Autodesk Fusion 360 part; units mm, degrees
(part 2 of 4)
  spline S9 degree 5 poles (-4.69563, -13.417878) (-4.69084, -13.420961) (-4.681355, -13.42726) (-4.667416, -13.437105) (-4.649379, -13.450989) (-4.627583, -13.469387) (-4.606332, -13.48855) (-4.58542, -13.508202) (-4.564695, -13.528137) (-4.544101, -13.548273) (-4.523643, -13.568609) (-4.503366, -13.589197) (-4.483326, -13.610104) (-4.463562, -13.631378) (-4.444078, -13.65302) (-4.424855, -13.675002) (-4.405861, -13.697281) (-4.387063, -13.71981) (-4.368435, -13.742557) (-4.349971, -13.765508) (-4.331672, -13.788665) (-4.313547, -13.812036) (-4.295604, -13.835631) (-4.27785, -13.859454) (-4.260283, -13.883502) (-4.242898, -13.907768) (-4.225689, -13.93224) (-4.208647, -13.956907) (-4.191769, -13.981763) (-4.175051, -14.006801) (-4.158495, -14.032021) (-4.1421, -14.057422) (-4.125867, -14.083003) (-4.109797, -14.108764) (-4.093889, -14.134702) (-4.078141, -14.160813) (-4.062552, -14.187093) (-4.047119, -14.213539) (-4.031842, -14.240149) (-4.016718, -14.266918) (-4.001749, -14.293845) (-3.986933, -14.32093) (-3.972271, -14.348169) (-3.957762, -14.375562) (-3.943405, -14.403106) (-3.9292, -14.4308) (-3.915146, -14.458641) (-3.901243, -14.486627) (-3.887491, -14.514757) (-3.873888, -14.543029) (-3.860434, -14.57144) (-3.84713, -14.599991) (-3.833974, -14.628678) (-3.820967, -14.657502) (-3.808109, -14.686459) (-3.795398, -14.715549) (-3.782836, -14.74477) (-3.770421, -14.774121) (-3.758153, -14.8036) (-3.746033, -14.833206) (-3.73406, -14.862938) (-3.722233, -14.892795) (-3.710553, -14.922775) (-3.69902, -14.952876) (-3.687633, -14.983098) (-3.676392, -15.01344) (-3.665298, -15.043899) (-3.65435, -15.074474) (-3.643548, -15.105165) (-3.632893, -15.135971) (-3.622383, -15.16689) (-3.614091, -15.191717) (-3.607937, -15.210388) (-3.603864, -15.222858) (-3.601835, -15.229098) knots 0 0 0 0 0 0 0.01428571 0.02857143 0.04285714 0.05714286 0.07142857 0.08571429 0.1 0.11428571 0.12857143 0.14285714 0.15714286 0.17142857 0.18571429 0.2 0.21428571 0.22857143 0.24285714 0.25714286 0.27142857 0.28571429 0.3 0.31428571 0.32857143 0.34285714 0.35714286 0.37142857 0.38571429 0.4 0.41428571 0.42857143 0.44285714 0.45714286 0.47142857 0.48571429 0.5 0.51428571 0.52857143 0.54285714 0.55714286 0.57142857 0.58571429 0.6 0.61428571 0.62857143 0.64285714 0.65714286 0.67142857 0.68571429 0.7 0.71428571 0.72857143 0.74285714 0.75714286 0.77142857 0.78571429 0.8 0.81428571 0.82857143 0.84285714 0.85714286 0.87142857 0.88571429 0.9 0.91428571 0.92857143 0.94285714 0.95714286 0.97142857 0.98571429 1 1 1 1 1 1
  line L9 (-4.69563, -13.417878) -> (-4.967876, -13.242652)
  line L10 (-4.547342, -12.508165) -> (-4.258409, -12.654246)
  spline S10 degree 5 poles (-4.258409, -12.654246) (-4.253325, -12.656816) (-4.243091, -12.661807) (-4.227544, -12.668844) (-4.20644, -12.677371) (-4.17954, -12.686854) (-4.152256, -12.69548) (-4.124722, -12.703566) (-4.097038, -12.711347) (-4.069248, -12.718915) (-4.041354, -12.726263) (-4.013334, -12.733327) (-3.985159, -12.740026) (-3.956807, -12.746301) (-3.92828, -12.752148) (-3.899591, -12.757598) (-3.870763, -12.7627) (-3.841817, -12.767507) (-3.81277, -12.772056) (-3.78363, -12.776361) (-3.754396, -12.780419) (-3.725065, -12.784219) (-3.695634, -12.787748) (-3.666102, -12.791) (-3.636469, -12.793975) (-3.606742, -12.796684) (-3.576926, -12.799137) (-3.547025, -12.801346) (-3.517046, -12.80332) (-3.48699, -12.805062) (-3.456859, -12.806573) (-3.426653, -12.807854) (-3.396374, -12.808902) (-3.366023, -12.80972) (-3.335602, -12.810309) (-3.305112, -12.810672) (-3.274556, -12.810812) (-3.243936, -12.810733) (-3.213254, -12.810438) (-3.182513, -12.809929) (-3.151712, -12.809207) (-3.120855, -12.808273) (-3.089941, -12.807129) (-3.058973, -12.805775) (-3.027951, -12.804212) (-2.996877, -12.802443) (-2.965752, -12.800469) (-2.934579, -12.798291) (-2.903358, -12.795912) (-2.87209, -12.793331) (-2.840777, -12.79055) (-2.80942, -12.787571) (-2.77802, -12.784394) (-2.746578, -12.78102) (-2.715096, -12.77745) (-2.683575, -12.773685) (-2.652015, -12.769726) (-2.620418, -12.765575) (-2.588785, -12.761231) (-2.557117, -12.756696) (-2.525415, -12.751971) (-2.49368, -12.747056) (-2.461913, -12.741952) (-2.430114, -12.73666) (-2.398286, -12.731181) (-2.36643, -12.725515) (-2.334546, -12.719663) (-2.302635, -12.713626) (-2.270699, -12.707405) (-2.238738, -12.701) (-2.206753, -12.694411) (-2.181145, -12.688994) (-2.161928, -12.684849) (-2.149112, -12.682049) (-2.142703, -12.68064) knots 0 0 0 0 0 0 0.01428571 0.02857143 0.04285714 0.05714286 0.07142857 0.08571429 0.1 0.11428571 0.12857143 0.14285714 0.15714286 0.17142857 0.18571429 0.2 0.21428571 0.22857143 0.24285714 0.25714286 0.27142857 0.28571429 0.3 0.31428571 0.32857143 0.34285714 0.35714286 0.37142857 0.38571429 0.4 0.41428571 0.42857143 0.44285714 0.45714286 0.47142857 0.48571429 0.5 0.51428571 0.52857143 0.54285714 0.55714286 0.57142857 0.58571429 0.6 0.61428571 0.62857143 0.64285714 0.65714286 0.67142857 0.68571429 0.7 0.71428571 0.72857143 0.74285714 0.75714286 0.77142857 0.78571429 0.8 0.81428571 0.82857143 0.84285714 0.85714286 0.87142857 0.88571429 0.9 0.91428571 0.92857143 0.94285714 0.95714286 0.97142857 0.98571429 1 1 1 1 1 1
  arc A5 (-2.142703, -12.68064) -> (-1.961546, -12.203578) centre (-12.332883, -8.53815) ccw
  spline S11 degree 5 poles (-3.561505, -10.819006) (-3.555996, -10.820458) (-3.545029, -10.823518) (-3.52873, -10.828574) (-3.507285, -10.836204) (-3.480872, -10.846966) (-3.454739, -10.858624) (-3.428777, -10.870852) (-3.402906, -10.883408) (-3.377098, -10.896194) (-3.351357, -10.909213) (-3.32571, -10.922527) (-3.30019, -10.936218) (-3.27482, -10.950344) (-3.249602, -10.964906) (-3.224527, -10.979871) (-3.199578, -10.99519) (-3.174738, -11.010808) (-3.149993, -11.026685) (-3.12534, -11.042808) (-3.100781, -11.059177) (-3.07632, -11.075803) (-3.051965, -11.092698) (-3.027718, -11.109869) (-3.00358, -11.127312) (-2.979547, -11.145017) (-2.955618, -11.162973) (-2.931787, -11.181168) (-2.908054, -11.199591) (-2.884418, -11.218238) (-2.860878, -11.237107) (-2.837436, -11.256198) (-2.814093, -11.275512) (-2.790849, -11.295046) (-2.767704, -11.314798) (-2.744659, -11.334764) (-2.721711, -11.354941) (-2.698861, -11.375324) (-2.676109, -11.39591) (-2.653454, -11.416696) (-2.630896, -11.43768) (-2.608436, -11.45886) (-2.586074, -11.480235) (-2.56381, -11.501804) (-2.541644, -11.523563) (-2.519576, -11.545512) (-2.497607, -11.567648) (-2.475737, -11.589968) (-2.453964, -11.612471) (-2.432291, -11.635156) (-2.410716, -11.658019) (-2.38924, -11.681061) (-2.367863, -11.704279) (-2.346586, -11.727673) (-2.325409, -11.751239) (-2.304331, -11.774978) (-2.283354, -11.798887) (-2.262476, -11.822965) (-2.2417, -11.84721) (-2.221024, -11.871622) (-2.200449, -11.896199) (-2.179975, -11.920939) (-2.159602, -11.945842) (-2.139332, -11.970907) (-2.119163, -11.996131) (-2.099096, -12.021514) (-2.079133, -12.047054) (-2.059272, -12.07275) (-2.039515, -12.098601) (-2.019862, -12.124606) (-2.000311, -12.150764) (-1.984754, -12.171813) (-1.973132, -12.187669) (-1.965404, -12.19827) (-1.961546, -12.203578) knots 0 0 0 0 0 0 0.01428571 0.02857143 0.04285714 0.05714286 0.07142857 0.08571429 0.1 0.11428571 0.12857143 0.14285714 0.15714286 0.17142857 0.18571429 0.2 0.21428571 0.22857143 0.24285714 0.25714286 0.27142857 0.28571429 0.3 0.31428571 0.32857143 0.34285714 0.35714286 0.37142857 0.38571429 0.4 0.41428571 0.42857143 0.44285714 0.45714286 0.47142857 0.48571429 0.5 0.51428571 0.52857143 0.54285714 0.55714286 0.57142857 0.58571429 0.6 0.61428571 0.62857143 0.64285714 0.65714286 0.67142857 0.68571429 0.7 0.71428571 0.72857143 0.74285714 0.75714286 0.77142857 0.78571429 0.8 0.81428571 0.82857143 0.84285714 0.85714286 0.87142857 0.88571429 0.9 0.91428571 0.92857143 0.94285714 0.95714286 0.97142857 0.98571429 1 1 1 1 1 1
  line L11 (-3.561505, -10.819006) -> (-3.874574, -10.736485)
  line L12 (-3.701592, -9.907995) -> (-3.381658, -9.95764)
  spline S12 degree 5 poles (-3.381658, -9.95764) (-3.376029, -9.958513) (-3.364753, -9.960098) (-3.347793, -9.961986) (-3.325087, -9.963574) (-3.296573, -9.96428) (-3.267959, -9.964053) (-3.239273, -9.963235) (-3.21054, -9.96208) (-3.181772, -9.96069) (-3.152972, -9.959058) (-3.12414, -9.957119) (-3.095274, -9.954783) (-3.066371, -9.951989) (-3.037433, -9.948735) (-3.008465, -9.945053) (-2.979471, -9.940997) (-2.950456, -9.936624) (-2.921425, -9.931975) (-2.892381, -9.927064) (-2.863323, -9.921889) (-2.834254, -9.91644) (-2.805173, -9.910702) (-2.776081, -9.904668) (-2.74698, -9.898341) (-2.71787, -9.891731) (-2.688755, -9.88485) (-2.659636, -9.877711) (-2.630513, -9.870324) (-2.60139, -9.862693) (-2.572267, -9.854819) (-2.543144, -9.846703) (-2.514023, -9.838344) (-2.484905, -9.829743) (-2.45579, -9.820902) (-2.42668, -9.811825) (-2.397577, -9.802516) (-2.36848, -9.792979) (-2.339391, -9.783217) (-2.310311, -9.773233) (-2.281242, -9.763029) (-2.252183, -9.752605) (-2.223136, -9.741964) (-2.194101, -9.731106) (-2.165081, -9.720034) (-2.136074, -9.708749) (-2.107083, -9.697254) (-2.078108, -9.685549) (-2.049151, -9.673638) (-2.020211, -9.661522) (-1.99129, -9.649201) (-1.962388, -9.636678) (-1.933507, -9.623953) (-1.904647, -9.611028) (-1.875808, -9.597904) (-1.846993, -9.584583) (-1.818201, -9.571065) (-1.789434, -9.557353) (-1.760691, -9.543447) (-1.731975, -9.529348) (-1.703284, -9.515057) (-1.674621, -9.500576) (-1.645986, -9.485906) (-1.617379, -9.471046) (-1.588802, -9.456) (-1.560256, -9.440767) (-1.531741, -9.425349) (-1.503257, -9.409747) (-1.474807, -9.393961) (-1.44639, -9.377993) (-1.418006, -9.361843) (-1.395325, -9.348778) (-1.37833, -9.338897) (-1.367006, -9.332274) (-1.361346, -9.328954) knots 0 0 0 0 0 0 0.01428571 0.02857143 0.04285714 0.05714286 0.07142857 0.08571429 0.1 0.11428571 0.12857143 0.14285714 0.15714286 0.17142857 0.18571429 0.2 0.21428571 0.22857143 0.24285714 0.25714286 0.27142857 0.28571429 0.3 0.31428571 0.32857143 0.34285714 0.35714286 0.37142857 0.38571429 0.4 0.41428571 0.42857143 0.44285714 0.45714286 0.47142857 0.48571429 0.5 0.51428571 0.52857143 0.54285714 0.55714286 0.57142857 0.58571429 0.6 0.61428571 0.62857143 0.64285714 0.65714286 0.67142857 0.68571429 0.7 0.71428571 0.72857143 0.74285714 0.75714286 0.77142857 0.78571429 0.8 0.81428571 0.82857143 0.84285714 0.85714286 0.87142857 0.88571429 0.9 0.91428571 0.92857143 0.94285714 0.95714286 0.97142857 0.98571429 1 1 1 1 1 1
  arc A6 (-1.361346, -9.328954) -> (-1.336476, -8.819259) centre (-12.332883, -8.53815) ccw
  spline S13 degree 5 poles (-3.285983, -7.996868) (-3.280296, -7.996547) (-3.26892, -7.996068) (-3.251856, -7.995839) (-3.229103, -7.99647) (-3.200656, -7.998543) (-3.1722, -8.001555) (-3.14373, -8.005162) (-3.115246, -8.009108) (-3.086749, -8.013293) (-3.058246, -8.01772) (-3.02974, -8.022458) (-3.001238, -8.027593) (-2.972744, -8.033187) (-2.944261, -8.039244) (-2.915788, -8.045728) (-2.887327, -8.052588) (-2.858876, -8.059765) (-2.830436, -8.067218) (-2.802007, -8.074933) (-2.773592, -8.082912) (-2.745191, -8.091166) (-2.716807, -8.099708) (-2.688441, -8.108546) (-2.660093, -8.117676) (-2.631766, -8.127088) (-2.603458, -8.136771) (-2.575172, -8.146711) (-2.546908, -8.156898) (-2.518666, -8.167329) (-2.490447, -8.178) (-2.462253, -8.188913) (-2.434084, -8.200068) (-2.405942, -8.211463) (-2.377826, -8.223096) (-2.349738, -8.234964) (-2.321679, -8.247062) (-2.293649, -8.259387) (-2.265649, -8.271934) (-2.237679, -8.284702) (-2.209741, -8.297688) (-2.181835, -8.310891) (-2.153962, -8.32431) (-2.126123, -8.337942) (-2.098318, -8.351787) (-2.070548, -8.365843) (-2.042814, -8.380106) (-2.015116, -8.394576) (-1.987456, -8.409249) (-1.959833, -8.424126) (-1.932249, -8.439204) (-1.904704, -8.454481) (-1.877198, -8.469958) (-1.849734, -8.485631) (-1.82231, -8.5015) (-1.794928, -8.517563) (-1.767589, -8.53382) (-1.740294, -8.550268) (-1.713042, -8.566906) (-1.685834, -8.583734) (-1.658671, -8.60075) (-1.631554, -8.617952) (-1.604483, -8.635341) (-1.577459, -8.652915) (-1.550483, -8.670672) (-1.523555, -8.688612) (-1.496676, -8.706733) (-1.469847, -8.725034) (-1.443069, -8.743514) (-1.416341, -8.762173) (-1.389664, -8.78101) (-1.368363, -8.796221) (-1.352411, -8.807709) (-1.341786, -8.815403) (-1.336476, -8.819259) knots 0 0 0 0 0 0 0.01428571 0.02857143 0.04285714 0.05714286 0.07142857 0.08571429 0.1 0.11428571 0.12857143 0.14285714 0.15714286 0.17142857 0.18571429 0.2 0.21428571 0.22857143 0.24285714 0.25714286 0.27142857 0.28571429 0.3 0.31428571 0.32857143 0.34285714 0.35714286 0.37142857 0.38571429 0.4 0.41428571 0.42857143 0.44285714 0.45714286 0.47142857 0.48571429 0.5 0.51428571 0.52857143 0.54285714 0.55714286 0.57142857 0.58571429 0.6 0.61428571 0.62857143 0.64285714 0.65714286 0.67142857 0.68571429 0.7 0.71428571 0.72857143 0.74285714 0.75714286 0.77142857 0.78571429 0.8 0.81428571 0.82857143 0.84285714 0.85714286 0.87142857 0.88571429 0.9 0.91428571 0.92857143 0.94285714 0.95714286 0.97142857 0.98571429 1 1 1 1 1 1
  line L13 (-3.285983, -7.996868) -> (-3.60923, -8.015129)
  line L14 (-3.700732, -7.173734) -> (-3.381116, -7.122084)
  spline S14 degree 5 poles (-3.381116, -7.122084) (-3.375492, -7.121176) (-3.364279, -7.119198) (-3.347565, -7.115753) (-3.325479, -7.110246) (-3.298143, -7.102107) (-3.270999, -7.093049) (-3.243971, -7.083406) (-3.217, -7.073429) (-3.19007, -7.063217) (-3.163184, -7.052766) (-3.136363, -7.042011) (-3.109631, -7.03087) (-3.083006, -7.019281) (-3.05649, -7.007244) (-3.030077, -6.99479) (-3.003756, -6.981973) (-2.977513, -6.968848) (-2.951339, -6.955456) (-2.925234, -6.94181) (-2.899198, -6.927909) (-2.873235, -6.913744) (-2.847351, -6.8993) (-2.821547, -6.884571) (-2.795825, -6.869561) (-2.770183, -6.85428) (-2.744619, -6.838738) (-2.719131, -6.822951) (-2.693717, -6.806926) (-2.668377, -6.790668) (-2.643112, -6.77418) (-2.617923, -6.757462) (-2.59281, -6.740513) (-2.567775, -6.723335) (-2.542817, -6.70593) (-2.517937, -6.688302) (-2.493134, -6.670455) (-2.468409, -6.652393) (-2.44376, -6.634121) (-2.419189, -6.615639) (-2.394695, -6.596951) (-2.37028, -6.578058) (-2.345943, -6.558961) (-2.321685, -6.539663) (-2.297506, -6.520165) (-2.273406, -6.500469) (-2.249387, -6.480577) (-2.225447, -6.460492) (-2.201587, -6.440215) (-2.177808, -6.419749) (-2.15411, -6.399094) (-2.130492, -6.378253) (-2.106957, -6.357226) (-2.083503, -6.336015) (-2.060132, -6.314622) (-2.036843, -6.293049) (-2.013638, -6.271295) (-1.990516, -6.249365) (-1.967477, -6.227257) (-1.944523, -6.204974) (-1.921653, -6.182517) (-1.898868, -6.159888) (-1.876167, -6.137086) (-1.853553, -6.114114) (-1.831024, -6.090974) (-1.808582, -6.067665) (-1.786226, -6.04419) (-1.763959, -6.020549) (-1.741779, -5.996745) (-1.719687, -5.972777) (-1.697682, -5.948646) (-1.680149, -5.929212) (-1.667039, -5.914563) (-1.658316, -5.904765) (-1.653959, -5.899857) knots 0 0 0 0 0 0 0.01428571 0.02857143 0.04285714 0.05714286 0.07142857 0.08571429 0.1 0.11428571 0.12857143 0.14285714 0.15714286 0.17142857 0.18571429 0.2 0.21428571 0.22857143 0.24285714 0.25714286 0.27142857 0.28571429 0.3 0.31428571 0.32857143 0.34285714 0.35714286 0.37142857 0.38571429 0.4 0.41428571 0.42857143 0.44285714 0.45714286 0.47142857 0.48571429 0.5 0.51428571 0.52857143 0.54285714 0.55714286 0.57142857 0.58571429 0.6 0.61428571 0.62857143 0.64285714 0.65714286 0.67142857 0.68571429 0.7 0.71428571 0.72857143 0.74285714 0.75714286 0.77142857 0.78571429 0.8 0.81428571 0.82857143 0.84285714 0.85714286 0.87142857 0.88571429 0.9 0.91428571 0.92857143 0.94285714 0.95714286 0.97142857 0.98571429 1 1 1 1 1 1
  arc A7 (-1.653959, -5.899857) -> (-1.78781, -5.407424) centre (-12.332883, -8.53815) ccw
  spline S15 degree 5 poles (-3.896035, -5.227714) (-3.890725, -5.225651) (-3.880054, -5.22168) (-3.863896, -5.21619) (-3.842062, -5.209759) (-3.814367, -5.20294) (-3.786373, -5.197011) (-3.758182, -5.191644) (-3.729872, -5.186595) (-3.701477, -5.181769) (-3.673, -5.177171) (-3.644426, -5.172868) (-3.615732, -5.168944) (-3.586904, -5.16546) (-3.557943, -5.162418) (-3.52886, -5.159787) (-3.499672, -5.157515) (-3.470396, -5.155549) (-3.441044, -5.153849) (-3.411623, -5.152402) (-3.382133, -5.15121) (-3.352572, -5.150283) (-3.322937, -5.149636) (-3.293228, -5.149275) (-3.263447, -5.149199) (-3.233597, -5.149397) (-3.203683, -5.149858) (-3.17371, -5.150571) (-3.143681, -5.151525) (-3.113598, -5.152718) (-3.083463, -5.154147) (-3.053276, -5.155814) (-3.023039, -5.157717) (-2.992753, -5.159858) (-2.962418, -5.162234) (-2.932038, -5.164842) (-2.901613, -5.167677) (-2.871147, -5.170736) (-2.840639, -5.174017) (-2.810093, -5.177517) (-2.77951, -5.181234) (-2.74889, -5.185167) (-2.718234, -5.189316) (-2.687545, -5.193679) (-2.656822, -5.198254) (-2.626068, -5.20304) (-2.595284, -5.208035) (-2.56447, -5.213237) (-2.533629, -5.218645) (-2.502761, -5.224258) (-2.471868, -5.230074) (-2.44095, -5.236092) (-2.410008, -5.242311) (-2.379045, -5.24873) (-2.34806, -5.255348) (-2.317054, -5.262164) (-2.28603, -5.269176) (-2.254987, -5.276384) (-2.223927, -5.283787) (-2.192851, -5.291384) (-2.16176, -5.299173) (-2.130654, -5.307154) (-2.099535, -5.315326) (-2.068403, -5.323689) (-2.037259, -5.332241) (-2.006106, -5.340981) (-1.974943, -5.349909) (-1.943772, -5.359024) (-1.912593, -5.368325) (-1.881408, -5.377812) (-1.850216, -5.387483) (-1.825257, -5.395367) (-1.806535, -5.401363) (-1.794052, -5.405398) (-1.78781, -5.407424) knots 0 0 0 0 0 0 0.01428571 0.02857143 0.04285714 0.05714286 0.07142857 0.08571429 0.1 0.11428571 0.12857143 0.14285714 0.15714286 0.17142857 0.18571429 0.2 0.21428571 0.22857143 0.24285714 0.25714286 0.27142857 0.28571429 0.3 0.31428571 0.32857143 0.34285714 0.35714286 0.37142857 0.38571429 0.4 0.41428571 0.42857143 0.44285714 0.45714286 0.47142857 0.48571429 0.5 0.51428571 0.52857143 0.54285714 0.55714286 0.57142857 0.58571429 0.6 0.61428571 0.62857143 0.64285714 0.65714286 0.67142857 0.68571429 0.7 0.71428571 0.72857143 0.74285714 0.75714286 0.77142857 0.78571429 0.8 0.81428571 0.82857143 0.84285714 0.85714286 0.87142857 0.88571429 0.9 0.91428571 0.92857143 0.94285714 0.95714286 0.97142857 0.98571429 1 1 1 1 1 1
  line L15 (-3.896035, -5.227714) -> (-4.197818, -5.344971)
  line L16 (-4.544847, -4.573032) -> (-4.256835, -4.425143)
  spline S16 degree 5 poles (-4.256835, -4.425143) (-4.251767, -4.422541) (-4.241714, -4.417195) (-4.226882, -4.408754) (-4.207579, -4.396692) (-4.184097, -4.380504) (-4.16108, -4.363501) (-4.138354, -4.345978) (-4.115787, -4.328155) (-4.09333, -4.31012) (-4.07099, -4.291873) (-4.048805, -4.273357) (-4.026824, -4.2545) (-4.005083, -4.235251) (-3.983585, -4.215609) (-3.962313, -4.195603) (-3.941241, -4.175279) (-3.920338, -4.154687) (-3.899584, -4.133862) (-3.878973, -4.112817) (-3.858507, -4.091551) (-3.838192, -4.070056) (-3.818038, -4.04832) (-3.798049, -4.026339) (-3.778224, -4.004115) (-3.758559, -3.981657) (-3.739049, -3.958977) (-3.719687, -3.936086) (-3.700469, -3.912992) (-3.681393, -3.8897) (-3.66246, -3.866211) (-3.64367, -3.842527) (-3.625024, -3.818648) (-3.606522, -3.794574) (-3.588164, -3.770308) (-3.569949, -3.745855) (-3.551875, -3.721217) (-3.533941, -3.696399) (-3.516146, -3.671403) (-3.498488, -3.646234) (-3.480968, -3.620891) (-3.463586, -3.595378) (-3.446341, -3.569696) (-3.429234, -3.543845) (-3.412264, -3.51783) (-3.39543, -3.491651) (-3.378733, -3.46531) (-3.362171, -3.43881) (-3.345745, -3.412153) (-3.329455, -3.38534) (-3.313299, -3.358373) (-3.297278, -3.331253) (-3.281392, -3.303983) (-3.265641, -3.276563) (-3.250024, -3.248995) (-3.234542, -3.22128) (-3.219194, -3.193421) (-3.203981, -3.165418) (-3.188902, -3.137274) (-3.173956, -3.108988) (-3.159145, -3.080563) (-3.144468, -3.052) (-3.129925, -3.0233) (-3.115516, -2.994464) (-3.10124, -2.965494) (-3.087099, -2.936391) (-3.073093, -2.907157) (-3.05922, -2.877792) (-3.045482, -2.848299) (-3.031877, -2.818677) (-3.018407, -2.788928) (-3.007737, -2.765026) (-2.999795, -2.747043) (-2.994528, -2.735029) (-2.9919, -2.729016) knots 0 0 0 0 0 0 0.01428571 0.02857143 0.04285714 0.05714286 0.07142857 0.08571429 0.1 0.11428571 0.12857143 0.14285714 0.15714286 0.17142857 0.18571429 0.2 0.21428571 0.22857143 0.24285714 0.25714286 0.27142857 0.28571429 0.3 0.31428571 0.32857143 0.34285714 0.35714286 0.37142857 0.38571429 0.4 0.41428571 0.42857143 0.44285714 0.45714286 0.47142857 0.48571429 0.5 0.51428571 0.52857143 0.54285714 0.55714286 0.57142857 0.58571429 0.6 0.61428571 0.62857143 0.64285714 0.65714286 0.67142857 0.68571429 0.7 0.71428571 0.72857143 0.74285714 0.75714286 0.77142857 0.78571429 0.8 0.81428571 0.82857143 0.84285714 0.85714286 0.87142857 0.88571429 0.9 0.91428571 0.92857143 0.94285714 0.95714286 0.97142857 0.98571429 1 1 1 1 1 1
  arc A8 (-2.9919, -2.729016) -> (-3.27137, -2.302046) centre (-12.332883, -8.53815) ccw
  spline S17 degree 5 poles (-5.331945, -2.782609) (-5.327532, -2.779006) (-5.318611, -2.771932) (-5.30494, -2.761718) (-5.286162, -2.748854) (-5.261929, -2.73381) (-5.237137, -2.719521) (-5.211985, -2.705705) (-5.186621, -2.692155) (-5.161107, -2.678791) (-5.135444, -2.665618) (-5.109598, -2.652696) (-5.083521, -2.640097) (-5.057181, -2.627875) (-5.030578, -2.616032) (-5.003731, -2.604543) (-4.976674, -2.593363) (-4.949438, -2.582446) (-4.922048, -2.57176) (-4.894514, -2.561292) (-4.866836, -2.551044) (-4.839008, -2.541028) (-4.811023, -2.531255) (-4.78288, -2.521732) (-4.75458, -2.512456) (-4.72613, -2.50342) (-4.697538, -2.494615) (-4.668811, -2.48603) (-4.639957, -2.477659) (-4.610978, -2.469497) (-4.581876, -2.461544) (-4.552652, -2.453801) (-4.523306, -2.446268) (-4.493841, -2.438945) (-4.464257, -2.43183) (-4.434557, -2.424922) (-4.404746, -2.418217) (-4.374825, -2.411712) (-4.344797, -2.405405) (-4.314665, -2.399294) (-4.284429, -2.393378) (-4.254092, -2.387657) (-4.223655, -2.38213) (-4.193119, -2.376795) (-4.162487, -2.371653) (-4.131759, -2.366701) (-4.100938, -2.361939) (-4.070025, -2.357364) (-4.039022, -2.352977) (-4.007931, -2.348777) (-3.976752, -2.344761) (-3.945488, -2.34093) (-3.914139, -2.337284) (-3.882707, -2.33382) (-3.851193, -2.330539) (-3.819599, -2.327441) (-3.787926, -2.324523) (-3.756175, -2.321785) (-3.724348, -2.319228) (-3.692446, -2.31685) (-3.660469, -2.31465) (-3.628419, -2.312628) (-3.596298, -2.310784) (-3.564105, -2.309117) (-3.531843, -2.307627) (-3.499513, -2.306312) (-3.467117, -2.305174) (-3.434655, -2.30421) (-3.402128, -2.303421) (-3.369538, -2.302806) (-3.336884, -2.302365) (-3.31071, -2.302151) (-3.291051, -2.302068) (-3.277933, -2.302048) (-3.27137, -2.302046) knots 0 0 0 0 0 0 0.01428571 0.02857143 0.04285714 0.05714286 0.07142857 0.08571429 0.1 0.11428571 0.12857143 0.14285714 0.15714286 0.17142857 0.18571429 0.2 0.21428571 0.22857143 0.24285714 0.25714286 0.27142857 0.28571429 0.3 0.31428571 0.32857143 0.34285714 0.35714286 0.37142857 0.38571429 0.4 0.41428571 0.42857143 0.44285714 0.45714286 0.47142857 0.48571429 0.5 0.51428571 0.52857143 0.54285714 0.55714286 0.57142857 0.58571429 0.6 0.61428571 0.62857143 0.64285714 0.65714286 0.67142857 0.68571429 0.7 0.71428571 0.72857143 0.74285714 0.75714286 0.77142857 0.78571429 0.8 0.81428571 0.82857143 0.84285714 0.85714286 0.87142857 0.88571429 0.9 0.91428571 0.92857143 0.94285714 0.95714286 0.97142857 0.98571429 1 1 1 1 1 1
  line L17 (-5.331945, -2.782609) -> (-5.582723, -2.987383)
  line L18 (-6.151309, -2.360463) -> (-5.923094, -2.130812)
  spline S18 degree 5 poles (-5.923094, -2.130812) (-5.919078, -2.126771) (-5.911169, -2.11858) (-5.899672, -2.105969) (-5.885041, -2.088533) (-5.86771, -2.06588) (-5.851074, -2.042597) (-5.834875, -2.018909) (-5.81892, -1.994985) (-5.803136, -1.970893) (-5.787528, -1.946635) (-5.77215, -1.922169) (-5.757073, -1.897443) (-5.742344, -1.872418) (-5.727968, -1.847094) (-5.713919, -1.821494) (-5.700158, -1.795653) (-5.686642, -1.769609) (-5.673339, -1.74339) (-5.66024, -1.717006) (-5.647347, -1.690457) (-5.634669, -1.663736) (-5.622218, -1.636836) (-5.61, -1.609754) (-5.598013, -1.582491) (-5.58625, -1.555056) (-5.574703, -1.527457) (-5.563363, -1.499703) (-5.552222, -1.4718) (-5.541277, -1.443753) (-5.530529, -1.415564) (-5.519977, -1.387233) (-5.509623, -1.35876) (-5.499466, -1.330147) (-5.489505, -1.301396) (-5.479738, -1.272511) (-5.470163, -1.243494) (-5.460776, -1.214348) (-5.451575, -1.185077) (-5.442559, -1.155683) (-5.433728, -1.126167) (-5.425081, -1.096531) (-5.416616, -1.066777) (-5.408335, -1.036905) (-5.400234, -1.006919) (-5.392314, -0.976819) (-5.384574, -0.946608) (-5.377012, -0.916287) (-5.369627, -0.885859) (-5.36242, -0.855324) (-5.355388, -0.824684) (-5.348531, -0.793942) (-5.34185, -0.763097) (-5.335343, -0.732151) (-5.32901, -0.701107) (-5.322849, -0.669964) (-5.316862, -0.638726) (-5.311046, -0.607393) (-5.305402, -0.575966) (-5.299929, -0.544446) (-5.294627, -0.512836) (-5.289495, -0.481135) (-5.284532, -0.449345) (-5.279739, -0.417468) (-5.275115, -0.385505) (-5.270659, -0.353456) (-5.266372, -0.321325) (-5.262252, -0.28911) (-5.2583, -0.256815) (-5.254515, -0.224439) (-5.250897, -0.191983) (-5.248136, -0.165955) (-5.24614, -0.146397) (-5.244842, -0.133343) (-5.244202, -0.126812) knots 0 0 0 0 0 0 0.01428571 0.02857143 0.04285714 0.05714286 0.07142857 0.08571429 0.1 0.11428571 0.12857143 0.14285714 0.15714286 0.17142857 0.18571429 0.2 0.21428571 0.22857143 0.24285714 0.25714286 0.27142857 0.28571429 0.3 0.31428571 0.32857143 0.34285714 0.35714286 0.37142857 0.38571429 0.4 0.41428571 0.42857143 0.44285714 0.45714286 0.47142857 0.48571429 0.5 0.51428571 0.52857143 0.54285714 0.55714286 0.57142857 0.58571429 0.6 0.61428571 0.62857143 0.64285714 0.65714286 0.67142857 0.68571429 0.7 0.71428571 0.72857143 0.74285714 0.75714286 0.77142857 0.78571429 0.8 0.81428571 0.82857143 0.84285714 0.85714286 0.87142857 0.88571429 0.9 0.91428571 0.92857143 0.94285714 0.95714286 0.97142857 0.98571429 1 1 1 1 1 1
  arc A9 (-5.244202, -0.126812) -> (-5.641934, 0.192899) centre (-12.332883, -8.53815) ccw
  spline S19 degree 5 poles (-7.453155, -0.900897) (-7.450072, -0.896106) (-7.443773, -0.886621) (-7.433927, -0.872682) (-7.420044, -0.854645) (-7.401646, -0.83285) (-7.382483, -0.811599) (-7.362831, -0.790686) (-7.342896, -0.769962) (-7.32276, -0.749367) (-7.302424, -0.72891) (-7.281836, -0.708633) (-7.260929, -0.688592) (-7.239655, -0.668829) (-7.218013, -0.649345) (-7.196031, -0.630122) (-7.173752, -0.611128) (-7.151223, -0.592329) (-7.128476, -0.573702) (-7.105525, -0.555237) (-7.082367, -0.536939) (-7.058997, -0.518813) (-7.035402, -0.500871) (-7.011579, -0.483117) (-6.987531, -0.46555) (-6.963265, -0.448165) (-6.938793, -0.430955) (-6.914125, -0.413914) (-6.88927, -0.397035) (-6.864232, -0.380318) (-6.839012, -0.363761) (-6.813611, -0.347366) (-6.788029, -0.331134) (-6.762269, -0.315064) (-6.736331, -0.299156) (-6.71022, -0.283408) (-6.68394, -0.267819) (-6.657493, -0.252386) (-6.630884, -0.237108) (-6.604115, -0.221985) (-6.577187, -0.207016) (-6.550103, -0.1922) (-6.522864, -0.177538) (-6.495471, -0.163028) (-6.467927, -0.148671) (-6.440233, -0.134467) (-6.412392, -0.120413) (-6.384406, -0.10651) (-6.356276, -0.092757) (-6.328004, -0.079154) (-6.299592, -0.065701) (-6.271042, -0.052396) (-6.242354, -0.039241) (-6.213531, -0.026234) (-6.184574, -0.013375) (-6.155484, -0.000665) (-6.126262, 0.011898) (-6.096912, 0.024313) (-6.067433, 0.03658) (-6.037826, 0.0487) (-6.008095, 0.060674) (-5.978238, 0.0725) (-5.948258, 0.08418) (-5.918157, 0.095714) (-5.887934, 0.107101) (-5.857593, 0.118341) (-5.827134, 0.129435) (-5.796558, 0.140383) (-5.765868, 0.151185) (-5.735062, 0.161841) (-5.704143, 0.172351) (-5.679316, 0.180643) (-5.660645, 0.186796) (-5.648175, 0.190869) (-5.641934, 0.192899) knots 0 0 0 0 0 0 0.01428571 0.02857143 0.04285714 0.05714286 0.07142857 0.08571429 0.1 0.11428571 0.12857143 0.14285714 0.15714286 0.17142857 0.18571429 0.2 0.21428571 0.22857143 0.24285714 0.25714286 0.27142857 0.28571429 0.3 0.31428571 0.32857143 0.34285714 0.35714286 0.37142857 0.38571429 0.4 0.41428571 0.42857143 0.44285714 0.45714286 0.47142857 0.48571429 0.5 0.51428571 0.52857143 0.54285714 0.55714286 0.57142857 0.58571429 0.6 0.61428571 0.62857143 0.64285714 0.65714286 0.67142857 0.68571429 0.7 0.71428571 0.72857143 0.74285714 0.75714286 0.77142857 0.78571429 0.8 0.81428571 0.82857143 0.84285714 0.85714286 0.87142857 0.88571429 0.9 0.91428571 0.92857143 0.94285714 0.95714286 0.97142857 0.98571429 1 1 1 1 1 1
  line L19 (-7.453155, -0.900897) -> (-7.628381, -1.173143)
  line L20 (-8.362867, -0.752609) -> (-8.216787, -0.463675)
  spline S20 degree 5 poles (-8.216787, -0.463675) (-8.214217, -0.458591) (-8.209226, -0.448358) (-8.202189, -0.432811) (-8.193662, -0.411706) (-8.184179, -0.384807) (-8.175553, -0.357523) (-8.167467, -0.329988) (-8.159686, -0.302305) (-8.152118, -0.274515) (-8.14477, -0.24662) (-8.137706, -0.218601) (-8.131007, -0.190425) (-8.124732, -0.162073) (-8.118885, -0.133546) (-8.113435, -0.104858) (-8.108333, -0.076029) (-8.103526, -0.047084) (-8.098977, -0.018037) (-8.094672, 0.011104) (-8.090614, 0.040338) (-8.086814, 0.069668) (-8.083284, 0.099099) (-8.080033, 0.128632) (-8.077057, 0.158264) (-8.074349, 0.187991) (-8.071895, 0.217808) (-8.069686, 0.247708) (-8.067713, 0.277688) (-8.065971, 0.307744) (-8.06446, 0.337875) (-8.063179, 0.36808) (-8.06213, 0.398359) (-8.061313, 0.42871) (-8.060724, 0.459132) (-8.060361, 0.489622) (-8.060221, 0.520178) (-8.0603, 0.550798) (-8.060595, 0.581479) (-8.061104, 0.612221) (-8.061826, 0.643021) (-8.062759, 0.673879) (-8.063904, 0.704792) (-8.065258, 0.735761) (-8.066821, 0.766783) (-8.06859, 0.797857) (-8.070564, 0.828981) (-8.072741, 0.860155) (-8.075121, 0.891376) (-8.077702, 0.922643) (-8.080483, 0.953956) (-8.083462, 0.985313) (-8.086639, 1.016713) (-8.090013, 1.048155) (-8.093583, 1.079637) (-8.097348, 1.111159) (-8.101307, 1.142719) (-8.105458, 1.174315) (-8.109802, 1.205948) (-8.114337, 1.237616) (-8.119062, 1.269318) (-8.123977, 1.301053) (-8.129081, 1.332821) (-8.134373, 1.364619) (-8.139852, 1.396447) (-8.145518, 1.428304) (-8.15137, 1.460188) (-8.157407, 1.492098) (-8.163628, 1.524034) (-8.170033, 1.555995) (-8.176621, 1.58798) (-8.182039, 1.613588) (-8.186184, 1.632805) (-8.188984, 1.645621) (-8.190393, 1.65203) knots 0 0 0 0 0 0 0.01428571 0.02857143 0.04285714 0.05714286 0.07142857 0.08571429 0.1 0.11428571 0.12857143 0.14285714 0.15714286 0.17142857 0.18571429 0.2 0.21428571 0.22857143 0.24285714 0.25714286 0.27142857 0.28571429 0.3 0.31428571 0.32857143 0.34285714 0.35714286 0.37142857 0.38571429 0.4 0.41428571 0.42857143 0.44285714 0.45714286 0.47142857 0.48571429 0.5 0.51428571 0.52857143 0.54285714 0.55714286 0.57142857 0.58571429 0.6 0.61428571 0.62857143 0.64285714 0.65714286 0.67142857 0.68571429 0.7 0.71428571 0.72857143 0.74285714 0.75714286 0.77142857 0.78571429 0.8 0.81428571 0.82857143 0.84285714 0.85714286 0.87142857 0.88571429 0.9 0.91428571 0.92857143 0.94285714 0.95714286 0.97142857 0.98571429 1 1 1 1 1 1
  arc A10 (-8.190393, 1.65203) -> (-8.667455, 1.833188) centre (-12.332883, -8.53815) ccw
  spline S21 degree 5 poles (-10.052027, 0.233228) (-10.050575, 0.238737) (-10.047515, 0.249704) (-10.042459, 0.266004) (-10.034829, 0.287448) (-10.024066, 0.313862) (-10.012409, 0.339995) (-10.00018, 0.365956) (-9.987625, 0.391827) (-9.974839, 0.417636) (-9.96182, 0.443376) (-9.948506, 0.469023) (-9.934815, 0.494543) (-9.920689, 0.519913) (-9.906127, 0.545131) (-9.891161, 0.570206) (-9.875843, 0.595155) (-9.860225, 0.619996) (-9.844348, 0.644741) (-9.828225, 0.669394) (-9.811856, 0.693953) (-9.79523, 0.718413) (-9.778335, 0.742768) (-9.761164, 0.767015) (-9.743721, 0.791154) (-9.726016, 0.815186) (-9.70806, 0.839116) (-9.689865, 0.862946) (-9.671442, 0.886679) (-9.652795, 0.910316) (-9.633926, 0.933855) (-9.614835, 0.957297) (-9.595521, 0.98064) (-9.575987, 1.003884) (-9.556235, 1.027029) (-9.536268, 1.050075) (-9.516092, 1.073022) (-9.495709, 1.095872) (-9.475123, 1.118624) (-9.454337, 1.14128) (-9.433353, 1.163837) (-9.412173, 1.186297) (-9.390798, 1.20866) (-9.369229, 1.230924) (-9.34747, 1.253089) (-9.325521, 1.275157) (-9.303385, 1.297126) (-9.281065, 1.318997) (-9.258562, 1.340769) (-9.235877, 1.362443) (-9.213013, 1.384017) (-9.189972, 1.405493) (-9.166753, 1.42687) (-9.14336, 1.448147) (-9.119794, 1.469325) (-9.096055, 1.490402) (-9.072146, 1.51138) (-9.048068, 1.532257) (-9.023823, 1.553034) (-8.999411, 1.573709) (-8.974834, 1.594285) (-8.950094, 1.614758) (-8.925191, 1.635131) (-8.900126, 1.655402) (-8.874902, 1.675571) (-8.849519, 1.695637) (-8.823979, 1.715601) (-8.798283, 1.735461) (-8.772432, 1.755218) (-8.746427, 1.774872) (-8.720269, 1.794422) (-8.69922, 1.80998) (-8.683364, 1.821602) (-8.672763, 1.829329) (-8.667455, 1.833188) knots 0 0 0 0 0 0 0.01428571 0.02857143 0.04285714 0.05714286 0.07142857 0.08571429 0.1 0.11428571 0.12857143 0.14285714 0.15714286 0.17142857 0.18571429 0.2 0.21428571 0.22857143 0.24285714 0.25714286 0.27142857 0.28571429 0.3 0.31428571 0.32857143 0.34285714 0.35714286 0.37142857 0.38571429 0.4 0.41428571 0.42857143 0.44285714 0.45714286 0.47142857 0.48571429 0.5 0.51428571 0.52857143 0.54285714 0.55714286 0.57142857 0.58571429 0.6 0.61428571 0.62857143 0.64285714 0.65714286 0.67142857 0.68571429 0.7 0.71428571 0.72857143 0.74285714 0.75714286 0.77142857 0.78571429 0.8 0.81428571 0.82857143 0.84285714 0.85714286 0.87142857 0.88571429 0.9 0.91428571 0.92857143 0.94285714 0.95714286 0.97142857 0.98571429 1 1 1 1 1 1
  line L21 (-10.052027, 0.233228) -> (-10.134548, -0.079841)
  line L22 (-10.963038, 0.093142) -> (-10.913393, 0.413075)
  spline S22 degree 5 poles (-10.913393, 0.413075) (-10.912519, 0.418705) (-10.910935, 0.42998) (-10.909047, 0.446941) (-10.907459, 0.469647) (-10.906753, 0.49816) (-10.90698, 0.526775) (-10.907798, 0.55546) (-10.908952, 0.584193) (-10.910343, 0.612962) (-10.911974, 0.641761) (-10.913914, 0.670593) (-10.91625, 0.699459) (-10.919044, 0.728362) (-10.922298, 0.7573) (-10.92598, 0.786269) (-10.930036, 0.815263) (-10.934409, 0.844277) (-10.939058, 0.873308) (-10.943969, 0.902353) (-10.949144, 0.93141) (-10.954593, 0.960479) (-10.960331, 0.98956) (-10.966365, 1.018652) (-10.972692, 1.047754) (-10.979302, 1.076863) (-10.986183, 1.105978) (-10.993322, 1.135098) (-11.000709, 1.16422) (-11.00834, 1.193343) (-11.016214, 1.222467) (-11.02433, 1.251589) (-11.032689, 1.28071) (-11.04129, 1.309829) (-11.050131, 1.338943) (-11.059208, 1.368053) (-11.068517, 1.397157) (-11.078054, 1.426254) (-11.087816, 1.455342) (-11.097799, 1.484422) (-11.108004, 1.513492) (-11.118427, 1.542551) (-11.129069, 1.571598) (-11.139927, 1.600632) (-11.150999, 1.629653) (-11.162284, 1.658659) (-11.173779, 1.68765) (-11.185483, 1.716625) (-11.197395, 1.745583) (-11.209511, 1.774523) (-11.221832, 1.803444) (-11.234355, 1.832345) (-11.24708, 1.861227) (-11.260005, 1.890087) (-11.273129, 1.918925) (-11.28645, 1.94774) (-11.299967, 1.976532) (-11.31368, 2.0053) (-11.327586, 2.034042) (-11.341685, 2.062759) (-11.355976, 2.091449) (-11.370457, 2.120112) (-11.385127, 2.148747) (-11.399986, 2.177354) (-11.415033, 2.205931) (-11.430266, 2.234478) (-11.445684, 2.262993) (-11.461286, 2.291476) (-11.477072, 2.319926) (-11.49304, 2.348344) (-11.50919, 2.376728) (-11.522255, 2.399408) (-11.532135, 2.416404) (-11.538759, 2.427727) (-11.542079, 2.433387) knots 0 0 0 0 0 0 0.01428571 0.02857143 0.04285714 0.05714286 0.07142857 0.08571429 0.1 0.11428571 0.12857143 0.14285714 0.15714286 0.17142857 0.18571429 0.2 0.21428571 0.22857143 0.24285714 0.25714286 0.27142857 0.28571429 0.3 0.31428571 0.32857143 0.34285714 0.35714286 0.37142857 0.38571429 0.4 0.41428571 0.42857143 0.44285714 0.45714286 0.47142857 0.48571429 0.5 0.51428571 0.52857143 0.54285714 0.55714286 0.57142857 0.58571429 0.6 0.61428571 0.62857143 0.64285714 0.65714286 0.67142857 0.68571429 0.7 0.71428571 0.72857143 0.74285714 0.75714286 0.77142857 0.78571429 0.8 0.81428571 0.82857143 0.84285714 0.85714286 0.87142857 0.88571429 0.9 0.91428571 0.92857143 0.94285714 0.95714286 0.97142857 0.98571429 1 1 1 1 1 1
  arc A11 (-11.542079, 2.433387) -> (-12.051773, 2.458258) centre (-12.332883, -8.53815) ccw
  spline S23 degree 5 poles (-12.874165, 0.50875) (-12.874486, 0.514438) (-12.874965, 0.525814) (-12.875193, 0.542878) (-12.874563, 0.565631) (-12.87249, 0.594077) (-12.869478, 0.622534) (-12.865871, 0.651003) (-12.861925, 0.679488) (-12.85774, 0.707984) (-12.853313, 0.736488) (-12.848575, 0.764994) (-12.84344, 0.793495) (-12.837846, 0.821989) (-12.831789, 0.850473) (-12.825305, 0.878945) (-12.818445, 0.907407) (-12.811268, 0.935858) (-12.803815, 0.964298) (-12.796099, 0.992726) (-12.788121, 1.021142) (-12.779867, 1.049542) (-12.771325, 1.077927) (-12.762487, 1.106293) (-12.753357, 1.13464) (-12.743945, 1.162968) (-12.734262, 1.191275) (-12.724322, 1.219561) (-12.714135, 1.247826) (-12.703704, 1.276067) (-12.693033, 1.304286) (-12.68212, 1.33248) (-12.670965, 1.360649) (-12.65957, 1.388792) (-12.647937, 1.416907) (-12.636069, 1.444995) (-12.623971, 1.473054) (-12.611646, 1.501084) (-12.599099, 1.529085) (-12.586331, 1.557054) (-12.573345, 1.584992) (-12.560142, 1.612898) (-12.546723, 1.640771) (-12.53309, 1.668611) (-12.519245, 1.696416) (-12.50519, 1.724186) (-12.490927, 1.75192) (-12.476457, 1.779617) (-12.461783, 1.807278) (-12.446907, 1.834901) (-12.431829, 1.862485) (-12.416551, 1.89003) (-12.401075, 1.917535) (-12.385402, 1.945) (-12.369533, 1.972423) (-12.35347, 1.999805) (-12.337213, 2.027144) (-12.320765, 2.05444) (-12.304127, 2.081692) (-12.287299, 2.108899) (-12.270283, 2.136062) (-12.25308, 2.163179) (-12.235692, 2.19025) (-12.218118, 2.217274) (-12.200361, 2.244251) (-12.182421, 2.271179) (-12.1643, 2.298057) (-12.145999, 2.324886) (-12.127519, 2.351665) (-12.10886, 2.378392) (-12.090023, 2.405069) (-12.074812, 2.42637) (-12.063324, 2.442323) (-12.055629, 2.452948) (-12.051773, 2.458258) knots 0 0 0 0 0 0 0.01428571 0.02857143 0.04285714 0.05714286 0.07142857 0.08571429 0.1 0.11428571 0.12857143 0.14285714 0.15714286 0.17142857 0.18571429 0.2 0.21428571 0.22857143 0.24285714 0.25714286 0.27142857 0.28571429 0.3 0.31428571 0.32857143 0.34285714 0.35714286 0.37142857 0.38571429 0.4 0.41428571 0.42857143 0.44285714 0.45714286 0.47142857 0.48571429 0.5 0.51428571 0.52857143 0.54285714 0.55714286 0.57142857 0.58571429 0.6 0.61428571 0.62857143 0.64285714 0.65714286 0.67142857 0.68571429 0.7 0.71428571 0.72857143 0.74285714 0.75714286 0.77142857 0.78571429 0.8 0.81428571 0.82857143 0.84285714 0.85714286 0.87142857 0.88571429 0.9 0.91428571 0.92857143 0.94285714 0.95714286 0.97142857 0.98571429 1 1 1 1 1 1
  line L23 (-12.874165, 0.50875) -> (-12.855903, 0.185503)
  line L24 (-13.697299, 0.094002) -> (-13.748948, 0.413618)
  spline S24 degree 5 poles (-13.748948, 0.413618) (-13.749857, 0.419242) (-13.751835, 0.430455) (-13.75528, 0.447169) (-13.760786, 0.469254) (-13.768926, 0.49659) (-13.777984, 0.523734) (-13.787627, 0.550763) (-13.797604, 0.577733) (-13.807816, 0.604664) (-13.818267, 0.631549) (-13.829021, 0.65837) (-13.840163, 0.685102) (-13.851752, 0.711727) (-13.863789, 0.738243) (-13.876243, 0.764656) (-13.88906, 0.790978) (-13.902185, 0.817221) (-13.915577, 0.843394) (-13.929223, 0.8695) (-13.943123, 0.895536) (-13.957289, 0.921498) (-13.971733, 0.947383) (-13.986462, 0.973186) (-14.001471, 0.998908) (-14.016753, 1.02455) (-14.032294, 1.050114) (-14.048082, 1.075603) (-14.064107, 1.101017) (-14.080365, 1.126356) (-14.096852, 1.151621) (-14.113571, 1.17681) (-14.13052, 1.201923) (-14.147698, 1.226958) (-14.165103, 1.251916) (-14.182731, 1.276796) (-14.200578, 1.301599) (-14.21864, 1.326325) (-14.236912, 1.350973) (-14.255394, 1.375544) (-14.274082, 1.400038) (-14.292975, 1.424453) (-14.312071, 1.44879) (-14.33137, 1.473049) (-14.350868, 1.497227) (-14.370564, 1.521327) (-14.390456, 1.545347) (-14.410541, 1.569287) (-14.430818, 1.593146) (-14.451284, 1.616925) (-14.471939, 1.640624) (-14.49278, 1.664241) (-14.513807, 1.687776) (-14.535018, 1.71123) (-14.556411, 1.734601) (-14.577984, 1.75789) (-14.599737, 1.781095) (-14.621668, 1.804218) (-14.643776, 1.827256) (-14.666059, 1.85021) (-14.688515, 1.87308) (-14.711145, 1.895866) (-14.733947, 1.918566) (-14.756918, 1.941181) (-14.780059, 1.963709) (-14.803368, 1.986152) (-14.826843, 2.008507) (-14.850483, 2.030775) (-14.874288, 2.052955) (-14.898256, 2.075047) (-14.922387, 2.097051) (-14.941821, 2.114584) (-14.95647, 2.127694) (-14.966268, 2.136417) (-14.971176, 2.140774) knots 0 0 0 0 0 0 0.01428571 0.02857143 0.04285714 0.05714286 0.07142857 0.08571429 0.1 0.11428571 0.12857143 0.14285714 0.15714286 0.17142857 0.18571429 0.2 0.21428571 0.22857143 0.24285714 0.25714286 0.27142857 0.28571429 0.3 0.31428571 0.32857143 0.34285714 0.35714286 0.37142857 0.38571429 0.4 0.41428571 0.42857143 0.44285714 0.45714286 0.47142857 0.48571429 0.5 0.51428571 0.52857143 0.54285714 0.55714286 0.57142857 0.58571429 0.6 0.61428571 0.62857143 0.64285714 0.65714286 0.67142857 0.68571429 0.7 0.71428571 0.72857143 0.74285714 0.75714286 0.77142857 0.78571429 0.8 0.81428571 0.82857143 0.84285714 0.85714286 0.87142857 0.88571429 0.9 0.91428571 0.92857143 0.94285714 0.95714286 0.97142857 0.98571429 1 1 1 1 1 1
  arc A12 (-14.971176, 2.140774) -> (-15.463609, 2.006923) centre (-12.332883, -8.53815) ccw
  spline S25 degree 5 poles (-15.643318, -0.101302) (-15.645382, -0.095992) (-15.649353, -0.085321) (-15.654843, -0.069163) (-15.661274, -0.047329) (-15.668093, -0.019634) (-15.674022, 0.008361) (-15.679389, 0.036552) (-15.684438, 0.064861) (-15.689264, 0.093256) (-15.693862, 0.121733) (-15.698165, 0.150308) (-15.702088, 0.179001) (-15.705573, 0.207829) (-15.708615, 0.23679) (-15.711246, 0.265873) (-15.713518, 0.295061) (-15.715484, 0.324338) (-15.717183, 0.353689) (-15.718631, 0.38311) (-15.719823, 0.412601) (-15.72075, 0.442162) (-15.721397, 0.471796) (-15.721757, 0.501505) (-15.721834, 0.531286) (-15.721636, 0.561136) (-15.721175, 0.59105) (-15.720462, 0.621023) (-15.719508, 0.651053) (-15.718315, 0.681135) (-15.716886, 0.711271) (-15.715219, 0.741457) (-15.713315, 0.771694) (-15.711174, 0.801981) (-15.708799, 0.832315) (-15.706191, 0.862696) (-15.703356, 0.89312) (-15.700297, 0.923587) (-15.697016, 0.954094) (-15.693516, 0.98464) (-15.689799, 1.015224) (-15.685866, 1.045844) (-15.681717, 1.076499) (-15.677354, 1.107189) (-15.672779, 1.137911) (-15.667993, 1.168665) (-15.662998, 1.19945) (-15.657796, 1.230263) (-15.652388, 1.261104) (-15.646775, 1.291972) (-15.640959, 1.322866) (-15.634941, 1.353783) (-15.628722, 1.384725) (-15.622303, 1.415689) (-15.615685, 1.446674) (-15.608869, 1.477679) (-15.601857, 1.508704) (-15.594649, 1.539746) (-15.587246, 1.570806) (-15.579649, 1.601882) (-15.57186, 1.632973) (-15.563879, 1.664079) (-15.555706, 1.695199) (-15.547344, 1.726331) (-15.538792, 1.757474) (-15.530051, 1.788628) (-15.521123, 1.819791) (-15.512009, 1.850962) (-15.502708, 1.88214) (-15.493221, 1.913326) (-15.48355, 1.944518) (-15.475666, 1.969477) (-15.469669, 1.988199) (-15.465635, 2.000681) (-15.463609, 2.006923) knots 0 0 0 0 0 0 0.01428571 0.02857143 0.04285714 0.05714286 0.07142857 0.08571429 0.1 0.11428571 0.12857143 0.14285714 0.15714286 0.17142857 0.18571429 0.2 0.21428571 0.22857143 0.24285714 0.25714286 0.27142857 0.28571429 0.3 0.31428571 0.32857143 0.34285714 0.35714286 0.37142857 0.38571429 0.4 0.41428571 0.42857143 0.44285714 0.45714286 0.47142857 0.48571429 0.5 0.51428571 0.52857143 0.54285714 0.55714286 0.57142857 0.58571429 0.6 0.61428571 0.62857143 0.64285714 0.65714286 0.67142857 0.68571429 0.7 0.71428571 0.72857143 0.74285714 0.75714286 0.77142857 0.78571429 0.8 0.81428571 0.82857143 0.84285714 0.85714286 0.87142857 0.88571429 0.9 0.91428571 0.92857143 0.94285714 0.95714286 0.97142857 0.98571429 1 1 1 1 1 1
  line L25 (-15.643318, -0.101302) -> (-15.526062, -0.403085)
  line L26 (-16.298001, -0.750114) -> (-16.44589, -0.462101)
  spline S26 degree 5 poles (-16.44589, -0.462101) (-16.448492, -0.457033) (-16.453837, -0.44698) (-16.462279, -0.432149) (-16.474341, -0.412846) (-16.490529, -0.389363) (-16.507532, -0.366347) (-16.525055, -0.343621) (-16.542878, -0.321054) (-16.560912, -0.298597) (-16.57916, -0.276257) (-16.597676, -0.254071) (-16.616533, -0.232091) (-16.635782, -0.21035) (-16.655424, -0.188852) (-16.67543, -0.16758) (-16.695754, -0.146507) (-16.716346, -0.125604) (-16.737171, -0.104851) (-16.758216, -0.08424) (-16.779482, -0.063773) (-16.800977, -0.043459) (-16.822713, -0.023305) (-16.844694, -0.003316) (-16.866918, 0.016509) (-16.889376, 0.036174) (-16.912056, 0.055684) (-16.934947, 0.075046) (-16.958041, 0.094265) (-16.981333, 0.11334) (-17.004822, 0.132274) (-17.028506, 0.151064) (-17.052385, 0.16971) (-17.076459, 0.188211) (-17.100724, 0.206569) (-17.125178, 0.224784) (-17.149816, 0.242858) (-17.174634, 0.260792) (-17.19963, 0.278588) (-17.224799, 0.296245) (-17.250142, 0.313765) (-17.275655, 0.331147) (-17.301337, 0.348392) (-17.327187, 0.365499) (-17.353203, 0.38247) (-17.379382, 0.399303) (-17.405723, 0.416) (-17.432223, 0.432562) (-17.45888, 0.448988) (-17.485693, 0.465279) (-17.51266, 0.481435) (-17.539779, 0.497455) (-17.56705, 0.513341) (-17.59447, 0.529093) (-17.622038, 0.544709) (-17.649752, 0.560191) (-17.677612, 0.575539) (-17.705615, 0.590753) (-17.733759, 0.605832) (-17.762045, 0.620777) (-17.79047, 0.635588) (-17.819033, 0.650265) (-17.847733, 0.664808) (-17.876569, 0.679218) (-17.905539, 0.693493) (-17.934642, 0.707634) (-17.963876, 0.721641) (-17.993241, 0.735513) (-18.022734, 0.749252) (-18.052356, 0.762856) (-18.082105, 0.776327) (-18.106006, 0.786996) (-18.12399, 0.794938) (-18.136004, 0.800206) (-18.142017, 0.802833) knots 0 0 0 0 0 0 0.01428571 0.02857143 0.04285714 0.05714286 0.07142857 0.08571429 0.1 0.11428571 0.12857143 0.14285714 0.15714286 0.17142857 0.18571429 0.2 0.21428571 0.22857143 0.24285714 0.25714286 0.27142857 0.28571429 0.3 0.31428571 0.32857143 0.34285714 0.35714286 0.37142857 0.38571429 0.4 0.41428571 0.42857143 0.44285714 0.45714286 0.47142857 0.48571429 0.5 0.51428571 0.52857143 0.54285714 0.55714286 0.57142857 0.58571429 0.6 0.61428571 0.62857143 0.64285714 0.65714286 0.67142857 0.68571429 0.7 0.71428571 0.72857143 0.74285714 0.75714286 0.77142857 0.78571429 0.8 0.81428571 0.82857143 0.84285714 0.85714286 0.87142857 0.88571429 0.9 0.91428571 0.92857143 0.94285714 0.95714286 0.97142857 0.98571429 1 1 1 1 1 1
  arc A13 (-18.142017, 0.802833) -> (-18.568987, 0.523363) centre (-12.332883, -8.53815) ccw
  spline S27 degree 5 poles (-18.088424, -1.537212) (-18.092027, -1.532799) (-18.099101, -1.523877) (-18.109315, -1.510206) (-18.122179, -1.491428) (-18.137223, -1.467196) (-18.151512, -1.442404) (-18.165328, -1.417251) (-18.178878, -1.391887) (-18.192242, -1.366374) (-18.205415, -1.340711) (-18.218337, -1.314865) (-18.230936, -1.288788) (-18.243158, -1.262448) (-18.255001, -1.235844) (-18.26649, -1.208998) (-18.27767, -1.18194) (-18.288587, -1.154705) (-18.299273, -1.127315) (-18.309741, -1.099781) (-18.319989, -1.072102) (-18.330005, -1.044274) (-18.339778, -1.01629) (-18.349301, -0.988147) (-18.358577, -0.959847) (-18.367613, -0.931397) (-18.376418, -0.902804) (-18.385002, -0.874078) (-18.393374, -0.845224) (-18.401536, -0.816244) (-18.409489, -0.787143) (-18.417232, -0.757919) (-18.424765, -0.728573) (-18.432088, -0.699107) (-18.439202, -0.669523) (-18.446111, -0.639824) (-18.452816, -0.610012) (-18.459321, -0.580092) (-18.465628, -0.550064) (-18.471739, -0.519931) (-18.477655, -0.489696) (-18.483376, -0.459359) (-18.488903, -0.428922) (-18.494238, -0.398386) (-18.49938, -0.367753) (-18.504332, -0.337026) (-18.509094, -0.306204) (-18.513668, -0.275292) (-18.518055, -0.244289) (-18.522256, -0.213197) (-18.526272, -0.182019) (-18.530102, -0.150754) (-18.533749, -0.119405) (-18.537213, -0.087973) (-18.540493, -0.05646) (-18.543592, -0.024866) (-18.54651, 0.006807) (-18.549247, 0.038558) (-18.551805, 0.070385) (-18.554183, 0.102288) (-18.556383, 0.134264) (-18.558405, 0.166314) (-18.560249, 0.198436) (-18.561916, 0.230628) (-18.563406, 0.26289) (-18.564721, 0.29522) (-18.565859, 0.327616) (-18.566823, 0.360079) (-18.567612, 0.392605) (-18.568227, 0.425196) (-18.568668, 0.45785) (-18.568882, 0.484024) (-18.568965, 0.503682) (-18.568985, 0.516801) (-18.568987, 0.523363) knots 0 0 0 0 0 0 0.01428571 0.02857143 0.04285714 0.05714286 0.07142857 0.08571429 0.1 0.11428571 0.12857143 0.14285714 0.15714286 0.17142857 0.18571429 0.2 0.21428571 0.22857143 0.24285714 0.25714286 0.27142857 0.28571429 0.3 0.31428571 0.32857143 0.34285714 0.35714286 0.37142857 0.38571429 0.4 0.41428571 0.42857143 0.44285714 0.45714286 0.47142857 0.48571429 0.5 0.51428571 0.52857143 0.54285714 0.55714286 0.57142857 0.58571429 0.6 0.61428571 0.62857143 0.64285714 0.65714286 0.67142857 0.68571429 0.7 0.71428571 0.72857143 0.74285714 0.75714286 0.77142857 0.78571429 0.8 0.81428571 0.82857143 0.84285714 0.85714286 0.87142857 0.88571429 0.9 0.91428571 0.92857143 0.94285714 0.95714286 0.97142857 0.98571429 1 1 1 1 1 1
  line L27 (-18.088424, -1.537212) -> (-17.88365, -1.78799)
  line L28 (-18.51057, -2.356576) -> (-18.740221, -2.12836)